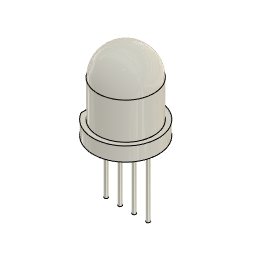
Individually Addressable RGB LED (Autodesk Fusion 360 design; units mm, degrees)
Autodesk Fusion 360 part; units mm, degrees
note: some values were not read from the file. Set by a fixed rule: which sketch regions a step uses.
sketch "Sketch1" plane through (0, 0, 0) normal (0, 0, 1) x (1, 0, 0)
  circle A0 centre (0, 0) radius 4.65
  circle A1 centre (0, 0) radius 4
  line L0 (-4, 2.3712) -> (-4, -2.3712)
  point P0 (-4, 0)
  dimension "d1" = 9.3
  dimension "d2" = 8
  constraint coincident A0.centre A1.centre
  constraint concentric A0 A1
  constraint coincident A0 L0.start
  constraint vertical L0
  constraint coincident A0 L0.end
  constraint coincident A1 P0
  constraint coincident L0 P0
  measures "d1" diameter of A0
  measures "d2" diameter of A1
extrude "Extrude1" add sketch "Sketch1" along normal blind 2 contours A1 | A0 L0 | A0 L0 makes body 1
extrude "Extrude2" add sketch "Sketch1" along normal blind 9.2 from surface at 2 contours A1 bodies 1
extrude "Extrude3" cut sketch "Sketch1" along normal up to surface (2 mm away) contours A0 L0 picked at (-4.4195, 0.2067) bodies 1
fillet "Fillet1" radius 4 1 edges at (-3.7293, -1.4465, 11.2) on bodies 1
sketch "Sketch2" plane through (0, 0, 0) normal (0, 0, 1) x (1, 0, 0)
  circle A0 centre (-2.7975, 0) radius 0.25
  circle A1 centre (-0.7975, 0) radius 0.25
  circle A2 centre (1.2025, 0) radius 0.25
  circle A3 centre (3.2025, 0) radius 0.25
  circle A4 centre (0, 0) radius 4 construction
  point P0 (-4, 0)
  dimension "d12" = 0.5
  dimension "d15" = 2
  dimension "d16" = 0
  measures "d12" diameter of A0
extrude "Extrude4" add sketch "Sketch2" against normal blind 9 separate body makes body 2 at (1.4522, -0.0125, -6) makes body 3 at (3.4522, -0.0125, -6) makes body 4 at (-0.5478, -0.0125, -6) makes body 5 at (-2.5478, -0.0125, -6)
equation "d7 = 11.2 mm - 2 mm"
